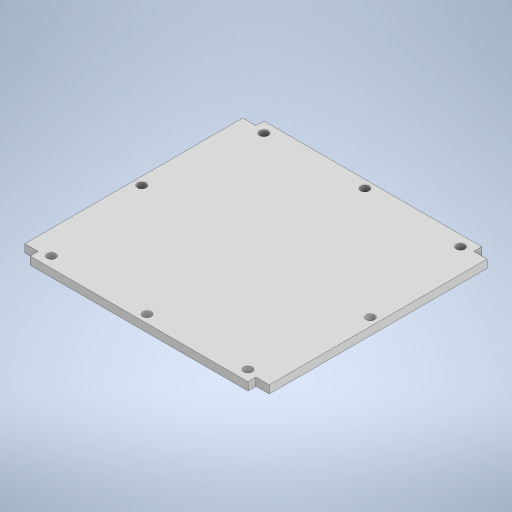
# Autodesk Inventor part: DummyUpperBoard
Saved by Autodesk Inventor 2023 (Build 270158000, 158)
## iProperties
Created: 2022-08-17
Part Number: DummyUpperBoard
Material: Generic
Document SubType Name: Modeling
Designer: Aditya Bansal
Density: 1 g/cm^3
Appearance: Default
Author: Aditya Bansal
Autodesk Inventor part; units mm, degrees
ref_plane "YZ Plane" through (0, 0, 0) normal (1, 0, 0) x (0, 1, 0)
ref_plane "XZ Plane" through (0, 0, 0) normal (0, 1, 0) x (-1, 0, 0)
ref_plane "XY Plane" through (0, 0, 0) normal (0, 0, 1) x (1, 0, 0)
sketch "Sketch1" plane through (0, 0, 0) normal (0, 1, 0) x (-1, 0, 0)
  line L0 (0, 0) -> (-92, 0)
  line L1 (-92, 0) -> (-92, -88)
  line L2 (-92, -88) -> (0, -88)
  line L3 (0, -88) -> (0, 0)
  line L4 (0, -88) -> (-5, -88)
  line L5 (-5, -88) -> (-5, -85)
  line L6 (-5, -85) -> (0, -85)
  line L7 (0, -85) -> (0, -88)
  line L8 (0, 0) -> (-5, 0)
  line L9 (-5, 0) -> (-5, -3)
  line L10 (-5, -3) -> (0, -3)
  line L11 (0, -3) -> (0, 0)
  line L12 (-92, 0) -> (-87, 0)
  line L13 (-87, 0) -> (-87, -3)
  line L14 (-87, -3) -> (-92, -3)
  line L15 (-92, -3) -> (-92, 0)
  line L16 (-92, -88) -> (-87, -88)
  line L17 (-87, -88) -> (-87, -85)
  line L18 (-87, -85) -> (-92, -85)
  line L19 (-92, -85) -> (-92, -88)
  circle A0 centre (-9, -84) radius 1.6
  circle A1 centre (-83, -84) radius 1.6
  circle A2 centre (-9, -4) radius 1.6
  circle A3 centre (-83, -4) radius 1.6
  circle A4 centre (-46, -85) radius 1.6
  circle A5 centre (-3, -44) radius 1.6
  circle A6 centre (-89, -44) radius 1.6
  circle A7 centre (-46, -3) radius 1.6
  point P0 (0, -85)
  point P1 (0, -3)
  dimension "d6" = 82
  dimension "d8" = 88
  dimension "d10" = 92
  dimension "d11" = 5
  dimension "d12" = 3.2
  dimension "d13" = 74
  dimension "d14" = 80
  dimension "d15" = 9
  dimension "d16" = 4
  dimension "d17" = 3.2
  dimension "d18" = 46
  dimension "d19" = 44
  dimension "d20" = 3
  dimension "d21" = 3
  dimension "d22" = 3
  dimension "d23" = 3
  constraints: 40 end point, 10 parallel, 8 centre point, 6 equal length, 6 equal radius, 5 horizontal, 5 perpendicular, 3 horizontal alignment, 3 vertical alignment, 1 point on line
  measures "d6" distance between parallel lines of L14 L18
  measures "d8" distance between parallel lines of L2 L0
  measures "d10" distance between parallel lines of L3 L1
  measures "d11" distance of L17.end L18.end
  measures "d12" diameter of A0
  measures "d13" distance of A1.centre A0.centre
  measures "d14" distance of A2.centre A0.centre
  measures "d15" distance from line of A0.centre L3
  measures "d16" distance from line of L0 A2.centre
  measures "d17" diameter of A7
  measures "d18" distance from line of L1 A7.centre
  measures "d19" distance from line of L2 A6.centre
  measures "d20" distance from line of L0 A7.centre
  measures "d21" distance from line of L2 A4.centre
  measures "d22" distance from line of L1 A6.centre
  measures "d23" distance from line of L3 A5.centre
extrude "Extrusion1" add sketch "Sketch1" along normal blind 3 contours L9 L10 L3 L6 L5 L2 L17 L18 L1 L14 L13 L0
equation "\"d15\" = -0.5 * d13 + 0.5 * d10"
equation "\"d16\" = -0.5 * d14 + 0.5 * d8"
equation "\"d18\" = 0.5 * d10"
equation "\"d19\" = 0.5 * d8"
equation "\"d21\" = d20"
equation "\"d23\" = d22"
body "Solid1"
